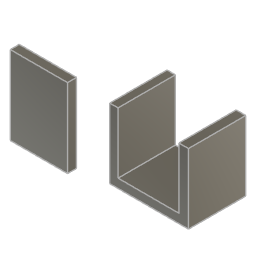
motor_bracket v1 (Autodesk Fusion 360 design; units mm, degrees)
Autodesk Fusion 360 part; units mm, degrees
sketch "Sketch1" plane through (0, 0, 0) normal (0, 1, 0) x (1, 0, 0)
  line L0 (0, -53.3233) -> (0, -10.1433)
  line L1 (0, -10.1433) -> (43.18, -10.1433)
  line L2 (43.18, -10.1433) -> (43.18, -53.3233)
  line L3 (43.18, -53.3233) -> (49.9793, -53.3233)
  line L4 (49.9793, -53.3233) -> (49.9793, -3.7933)
  line L5 (49.9793, -3.7933) -> (-5.9007, -3.7933)
  line L6 (-5.9007, -3.7933) -> (-5.9007, -53.3233)
  line L7 (-5.9007, -53.3233) -> (0, -53.3233)
  dimension "d1" = 43.18
  dimension "d2" = 43.18
  dimension "d3" = 43.18
  dimension "d4" = 49.53
  dimension "d5" = 55.88
  dimension "d6" = 49.53
  constraint vertical L0
  constraint perpendicular L0 L1
  constraint perpendicular L1 L2
  constraint perpendicular L2 L3
  constraint perpendicular L3 L4
  constraint perpendicular L4 L5
  constraint perpendicular L5 L6
  measures "d1" distance of L0.start L0.end
  measures "d2" distance of L0.end L1.end
  measures "d3" distance of L1.end L2.end
  measures "d4" distance of L3.end L4.end
  measures "d5" distance of L4.end L5.end
  measures "d6" distance of L5.end L6.end
extrude "Extrude1" add sketch "Sketch1" along normal blind 40.64 makes body 1
sketch "Sketch2" plane through (0, 0, 0) normal (0, 1, 0) x (1, 0, 0)
  line L0 (-76.4881, -50.9221) -> (-35.8481, -50.9221)
  line L1 (-35.8481, -50.9221) -> (-35.8481, 4.9579)
  line L2 (-35.8481, 4.9579) -> (-76.4881, 4.9579)
  line L3 (-76.4881, 4.9579) -> (-76.4881, -50.9221)
  dimension "d9" = 40.64
  dimension "d10" = 55.88
  constraint horizontal L0
  constraint vertical L1
  constraint horizontal L2
  constraint vertical L3
  measures "d9" distance of L0.start L0.end
  measures "d10" distance of L0.start L2.end
extrude "Extrude2" add sketch "Sketch2" along normal blind 6.35 separate body makes body 2
